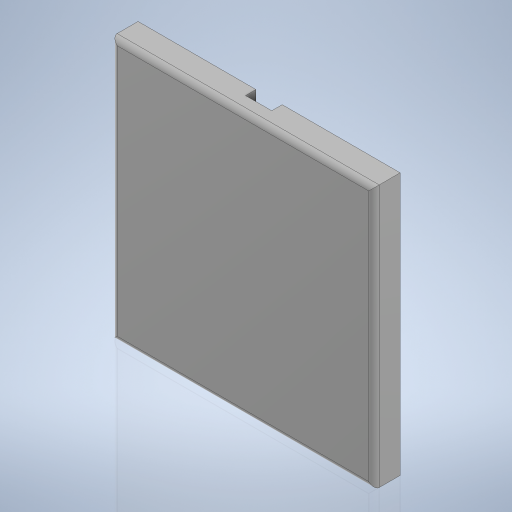
# Autodesk Inventor part: Tile
Saved by Autodesk Inventor 2023 (Build 270158000, 158)
## iProperties
Created: 2022-11-05
Part Number: Tile
Material: Acetalharz, Weiß
Document SubType Name: Modeling
Designer: RubenStein
Density: 1.425 g/cm^3
Appearance: Glatt - Weiß
Mass: 16.8984 g
Surface Area: 62.2847 cm^2
Volume: 11.8586 cm^3
Author: RubenStein
Autodesk Inventor part; units mm, degrees
ref_plane "YZ Plane" through (0, 0, 0) normal (1, 0, 0) x (0, 1, 0)
ref_plane "XZ Plane" through (0, 0, 0) normal (0, 1, 0) x (-1, 0, 0)
ref_plane "XY Plane" through (0, 0, 0) normal (0, 0, 1) x (1, 0, 0)
sketch "Skizze1" plane through (0, 0, 0) normal (0, 0, 1) x (1, 0, 0)
  line L0 (0, 0) -> (50, 0)
  line L1 (50, 0) -> (50, 50)
  line L2 (50, 50) -> (0, 50)
  line L3 (0, 50) -> (0, 0)
  dimension "d0" = 50
  constraints: 8 end point, 2 parallel, 2 perpendicular, 1 horizontal
  measures "d0" distance of L1.end L2.end
extrude "Extrusion1" add sketch "Skizze1" along normal blind 5
sketch "Skizze2" plane through (0, 0, 0) normal (0, 0, -1) x (-1, 0, 0)
  circle A0 centre (-25, 25) radius 4.55
  line L0 (0, 50) -> (0, 0) projected
  line L1 (0, 0) -> (-50, 0) projected
  dimension "d3" = 25
  dimension "d4" = 25
  dimension "d5" = 9.1
  constraints: 1 centre point
  measures "d3" distance from line of L0 A0.centre
  measures "d4" distance from line of L1 A0.centre
  measures "d5" diameter of A0
extrude "Extrusion2" cut sketch "Skizze2" against normal blind 3.5
sketch "Skizze3" plane through (0, 0, 0) normal (0, 0, -1) x (-1, 0, 0)
  circle A0 centre (-25, 25) radius 4.55 projected
  line L0 (-50, 50) -> (0, 50) projected
  line L1 (-22.5, 0) -> (-27.5, 0)
  line L2 (-27.5, 0) -> (-27.5, 50)
  line L3 (-27.5, 50) -> (-22.5, 50)
  line L4 (-22.5, 50) -> (-22.5, 0)
  line L5 (-22.5, 0) -> (-27.5, 50) construction
  line L6 (-27.5, 0) -> (-22.5, 50) construction
  point P0 (0, 0)
  dimension "d8" = 5
  constraints: 12 end point, 2 midpoint, 2 parallel, 1 horizontal, 1 perpendicular, 1 point on line
  measures "d8" distance between parallel lines of L4 L2
extrude "Extrusion3" cut sketch "Skizze3" against normal blind 2 contours L4 A0 L2 | A0 L2 L0 L4 | L4 L1 L2 A0
fillet "Rundung1" radius 1 4 edges at (0, 25, 5) (25, 50, 5) (50, 25, 5) (25, 0, 5)
